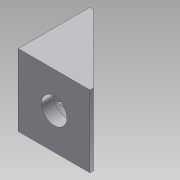
# Autodesk Inventor part: 90 Degree Corner Connector
Saved by Autodesk Inventor 2013 SP2 (Build 170200200, 200)
## iProperties
Created: 2013-06-26
Part Number: 90 Degree Corner Connector
Material: Acetal Resin, White
Document SubType Name: Modeling
Designer: Jon Hollander
Density: 1.425 g/cm^3
Mass: 4.58485 g
Surface Area: 20.962 cm^2
Volume: 3.21744 cm^3
Author: Jon Hollander
Autodesk Inventor part; units mm, degrees
ref_plane "YZ Plane" through (0, 0, 0) normal (1, 0, 0) x (0, 1, 0)
ref_plane "XZ Plane" through (0, 0, 0) normal (0, 1, 0) x (-1, 0, 0)
sketch "Sketch1" plane through (0, 0, 0) normal (0, 0, 1) x (1, 0, 0)
  line L0 (0, 0) -> (0, 20)
  line L1 (20, 0) -> (0, 0)
  line L2 (0, 20) -> (1, 20)
  line L3 (1, 20) -> (20, 1.0001)
  line L4 (20, 1.0001) -> (20, 0)
  dimension "d0" = 20
  dimension "d1" = 20
  dimension "d2" = 1
  dimension "d3" = 26.87
  dimension "d4" = 1.0001
  constraints: 10 end point, 2 perpendicular, 1 parallel, 1 vertical
  measures "d0" distance of L0.start L0.end
  measures "d1" distance of L1.start L0.start
  measures "d2" distance of L0.end L2.end
  measures "d3" distance of L2.end L3.end
  measures "d4" distance of L3.end L1.start
extrude "Extrusion1" add sketch "Sketch1" along normal blind 20
sketch "Sketch2" plane through (0, 0, 0) normal (-1, 0, 0) x (0, 0, 1)
  line L0 (0, 0) -> (20, 0) projected
  circle A0 centre (10, 10) radius 3.57
  circle A1 centre (10, 10) radius 5.5
  line L1 (10, 19.6278) -> (10, 0) construction
  dimension "d7" = 7.14
  dimension "d8" = 11
  dimension "d9" = 4.5
  constraints: 2 centre point, 2 end point, 1 coincident, 1 midpoint, 1 point on line
  measures "d7" diameter of A0
  measures "d8" diameter of A1
  measures "d9" distance edge to line of A1 L0
extrude "Extrusion2" cut sketch "Sketch2" against normal through all contours A0
sketch "Sketch3" plane through (0, 0, 0) normal (0, -1, 0) x (1, 0, 0)
  circle A0 centre (10, 10) radius 3.57
  dimension "d12" = 7.14
  constraints: 1 centre point
  measures "d12" diameter of A0
extrude "Extrusion3" cut sketch "Sketch3" against normal through all
ref_plane "Work Plane1" through (20, 1.0001, 20) normal (-1, 0, 0) x (0, 0, 1)
sketch "Sketch4" plane through (20, 1.0001, 20) normal (-1, 0, 0) x (0, 0, 1)
  circle A0 centre (-10, 8.9999) radius 3.57 projected
  circle A1 centre (-10, 8.9999) radius 5.5
  point P0 (-20, -1.0001)
  dimension "d15" = 11
  constraints: 1 centre point, 1 coincident
  measures "d15" diameter of A1
extrude "Extrusion4" cut sketch "Sketch4" along normal blind 16.5
sketch "Sketch5" plane through (0, 20, 0) normal (0, 1, 0) x (1, 0, 0)
  circle A0 centre (10, -10) radius 5.5
  dimension "d18" = 11
  constraints: 1 centre point, 1 coincident
  measures "d18" diameter of A0
extrude "Extrusion5" cut sketch "Sketch5" against normal blind 16.5
equation "\"d1\" = d0"
body "Solid1"
